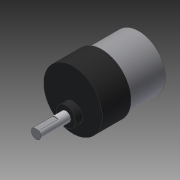
# Autodesk Inventor part: Drive Motor
Saved by Autodesk Inventor 2014 SP1 (Build 180222100, 222)
## iProperties
Created: 2014-01-12
Part Number: Drive Motor
Material: Generic
Document SubType Name: Modeling
Designer: tom
Density: 1 g/cm^3
Appearance: Default
d0: 1.425 in
d1: 0.700 in
d2: 0.00 deg
d3: 0.449 in
d4: 0.470 in
d5: 0.170 in
d6: 0.00 deg
d7: 0.236 in
d8: 0.725 in
d9: 0.00 deg
d11: 0.472 in
d12: 0.00 deg
d13: 1.300 in
d14: 0.900 in
d15: 0.00 deg
d16: 0.350 in
d17: 0.125 in
d18: 0.00 deg
d21: 0.118 in
d22: 0.118 in
d23: 2.114 in
d24: 2.114 in
d25: 0.118 in
d26: 0.118 in
d27: 0.500 in
d28: 0.00 deg
Author: tom
Autodesk Inventor part; units mm, degrees
ref_plane "YZ Plane" through (0, 0, 0) normal (1, 0, 0) x (0, 1, 0)
ref_plane "XZ Plane" through (0, 0, 0) normal (0, 1, 0) x (-1, 0, 0)
ref_plane "XY Plane" through (0, 0, 0) normal (0, 0, 1) x (1, 0, 0)
sketch "Sketch1" plane through (0, 0, 0) normal (0, 0, 1) x (1, 0, 0)
  circle A0 centre (0, 0) radius 18.0975
  dimension "d0" = 36.195
  constraints: 1 centre point, 1 coincident
  measures "d0" diameter of A0
extrude "Extrusion1" add sketch "Sketch1" along normal blind 17.78
sketch "Sketch2" plane through (0, 0, 17.78) normal (0, 0, 1) x (1, 0, 0)
  circle A0 centre (0, 0) radius 18.0975 projected
  line L0 (0, -18.0975) -> (0, -6.6929) construction
  circle A1 centre (0, -6.6929) radius 5.969
  dimension "d3" = 11.4046
  dimension "d4" = 11.938
  constraints: 2 end point, 1 centre point, 1 coincident, 1 vertical, 1 vertical alignment, 1 other
  measures "d3" distance of L0.start L0.end
  measures "d4" diameter of A1
extrude "Extrusion2" add sketch "Sketch2" along normal blind 4.318 contours A1
sketch "Sketch3" plane through (0, -6.6929, 22.098) normal (0, 0, 1) x (1, 0, 0)
  circle A0 centre (0, 0) radius 5.969 projected
  circle A1 centre (0, 0) radius 3
  point P0 (0, 6.6929)
  dimension "d7" = 6
  constraints: 1 centre point, 1 coincident
  measures "d7" diameter of A1
extrude "Extrusion3" add sketch "Sketch3" along normal blind 18.415 contours A1
sketch "Sketch4" plane through (0, -6.6929, 40.513) normal (0, 0, 1) x (1, 0, 0)
  circle A0 centre (0, 0) radius 3 projected
  arc A1 (1.6583, 2.5) -> (-1.6583, 2.5) centre (0, 0) ccw
  line L0 (-1.6583, 2.5) -> (1.6583, 2.5)
  point P0 (0, 6.6929)
  constraints: 2 end point, 2 point on circle, 1 centre point, 1 coincident
extrude "Extrusion4" cut sketch "Sketch4" against normal blind 12 contours L0 A0 picked at (-0.1169, 2.6598)
sketch "Sketch5" plane through (0, 0, 0) normal (0, 0, -1) x (-1, 0, 0)
  circle A0 centre (0, 0) radius 18.0975 projected
  circle A1 centre (0, 0) radius 16.51
  dimension "d13" = 33.02
  constraints: 1 centre point, 1 coincident
  measures "d13" diameter of A1
extrude "Extrusion5" add sketch "Sketch5" along normal blind 22.86 contours A1
sketch "Sketch6" plane through (0, 0, -22.86) normal (0, 0, -1) x (-1, 0, 0)
  circle A0 centre (0, 0) radius 16.51 projected
  circle A1 centre (0, 0) radius 4.445
  dimension "d16" = 8.89
  constraints: 1 centre point, 1 coincident
  measures "d16" diameter of A1
extrude "Extrusion6" add sketch "Sketch6" along normal blind 3.175 contours A1
sketch "Sketch7" plane through (0, 0, 17.78) normal (0, 0, 1) x (1, 0, 0)
  circle A0 centre (0, 0) radius 18.0975 projected
  circle A1 centre (-15.494, 0) radius 1.5
  circle A2 centre (15.494, 0) radius 1.5
  circle A3 centre (0, 0) radius 15.494 construction
  circle A4 centre (15.494, 0) radius 26.8478 construction
  circle A5 centre (-7.7668, 13.4068) radius 26.8478 construction
  circle A6 centre (-7.7668, 13.4068) radius 1.5
  circle A7 centre (-7.747, -13.441) radius 1.5
  dimension "d24" = 53.6956
  dimension "d21" = 3
  dimension "d22" = 3
  dimension "d23" = 53.6956
  dimension "d25" = 3
  dimension "d26" = 3
  constraints: 6 centre point, 4 point on circle, 3 coincident, 3 other
  measures "d21" diameter of A1
  measures "d22" diameter of A2
  measures "d23" diameter of A4
  measures "d25" diameter of A6
  measures "d26" diameter of A7
extrude "Extrusion7" cut sketch "Sketch7" against normal blind 12.7 contours A1 | A2 | A6 | A7
thread "Thread1" size "M3x0.5" class "6H" standard "ISO Metric profile" full length
thread "Thread2" size "5-40 UNC" class "2B" standard "ANSI Unified Screw Threads" full length
thread "Thread3" size "5-40 UNC" class "2B" standard "ANSI Unified Screw Threads" full length
thread "Thread4" size "5-40 UNC" class "2B" standard "ANSI Unified Screw Threads" full length
body "Solid1"
